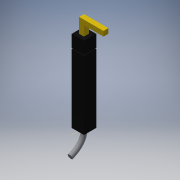
# Autodesk Inventor part: Pin-connector-angled
Saved by Autodesk Inventor 2016 (Build 200138000, 138)
## iProperties
Created: 2015-06-24
Part Number: Pin-connector-angled
Material: Generic
Document SubType Name: Modeling
Designer: Openlab
Density: 1 g/cm^3
Appearance: Default
Author: Openlab
Autodesk Inventor part; units mm, degrees
ref_plane "YZ Plane" through (0, 0, 0) normal (1, 0, 0) x (0, 1, 0)
ref_plane "XZ Plane" through (0, 0, 0) normal (0, 1, 0) x (-1, 0, 0)
sketch "Sketch1" plane through (0, 0, 0) normal (0, 1, 0) x (-1, 0, 0)
  line L0 (0, 0) -> (5, 0)
  line L1 (5, 0) -> (5, -13)
  line L2 (5, -13) -> (4, -13)
  line L3 (4, -13) -> (4, -1)
  line L4 (4, -1) -> (0, -1)
  line L5 (0, -1) -> (0, 0)
  line L6 (5.75, -3) -> (3.25, -3)
  line L7 (3.25, -3) -> (3.25, -5.5)
  line L8 (3.25, -5.5) -> (5.75, -5.5)
  line L9 (5.75, -5.5) -> (5.75, -3)
  line L10 (4.5, -1.8535) -> (4.5, -3.6396) construction
  line L11 (5.75, -5.7) -> (3.25, -5.7)
  line L12 (3.25, -5.7) -> (3.25, -19.7)
  line L13 (3.25, -19.7) -> (5.75, -19.7)
  line L14 (5.75, -19.7) -> (5.75, -5.7)
  dimension "d0" = 4
  dimension "d1" = 5
  dimension "d2" = 2.5
  dimension "d3" = 2.5
  dimension "d4" = 2
  dimension "d16" = 0.2
  dimension "d19" = 14
  dimension "d20" = 7.5
  constraints: 30 end point, 8 perpendicular, 2 collinear, 2 horizontal, 2 parallel, 1 vertical, 2 other
  measures "d0" distance between parallel lines of L5 L3
  measures "d1" distance between parallel lines of L5 L1
  measures "d2" distance of L8.end L6.start
  measures "d3" distance of L6.start L6.end
  measures "d4" distance between parallel lines of L6 L4
  measures "d16" distance between parallel lines of L11 L8
  measures "d19" distance between parallel lines of L13 L11
  measures "d20" distance between parallel lines of L2 L8
extrude "Extrusion1" add sketch "Sketch1" along normal blind 0.5 and the other way blind 0.5 contours L0 L1 L6 L3 L4 L5 | L1 L8 L3 L6 | L1 L11 L3 L8 | L1 L2 L3 L11
extrude "Extrusion2" add sketch "Sketch1" against normal blind 1.25 and the other way blind 1.25 contours L6 L9 L8 L1 | L1 L8 L3 L6 | L3 L8 L7 L6 | L11 L14 L13 L12 L3 L2 L1 | L1 L2 L3 L11
sketch "Sketch2" plane through (-3.25, -1.25, -19.7) normal (0, 0, -1) x (-1, 0, 0)
  line L0 (1.25, 3.4717) -> (1.25, -1.4422) construction
  constraints: 2 end point, 1 vertical
ref_plane "Work Plane1" through (-4.5, 2.2217, -19.7) normal (1, 0, 0) x (0, -1, 0)
sketch "Sketch3" plane through (-4.5, 2.2217, -19.7) normal (1, 0, 0) x (0, -1, 0)
  line L0 (2.2217, 0.0174) -> (2.2217, 2.5917) construction
  line L1 (2.2217, 2.5917) -> (5.0748, 3.6547) construction
  spline S0 degree 2 poles (2.2217, 0.0174) (2.2217, 2.5917) (5.0748, 3.6547) knots 1 1 1 2 2 2
  point P0 (2.2217, -19.7)
  constraints: 1 vertical, 3 other
sketch "Sketch4" plane through (-3.25, -1.25, -19.7) normal (0, 0, -1) x (-1, 0, 0)
  circle A0 centre (1.2535, 1.3137) radius 0.5
  point P0 (-3.25, 1.25)
  dimension "d22" = 1
  constraints: 1 centre point
  measures "d22" diameter of A0
sweep "Sweep1" add profiles "Sketch4" path "Sketch3"
body "Solid1"
